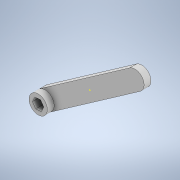
# Autodesk Inventor part: part
Saved by Autodesk Inventor 2020.2 (Build 242310000, 310)
## iProperties
Created: 2020-02-14
Part Number: part
Material: Generic
Document SubType Name: Modeling
Designer: robst
Density: 1 g/cm^3
Appearance: Default
Author: robst
Autodesk Inventor part; units mm, degrees
ref_plane "YZ Plane" through (0, 0, 0) normal (1, 0, 0) x (0, 1, 0)
ref_plane "XZ Plane" through (0, 0, 0) normal (0, 1, 0) x (-1, 0, 0)
ref_plane "XY Plane" through (0, 0, 0) normal (0, 0, 1) x (1, 0, 0)
sketch "Sketch1" plane through (0, 0, 0) normal (0, 0, 1) x (1, 0, 0)
  line L0 (-65.5382, -61.3942) -> (80.107, 40.5877)
  line L1 (80.107, 40.5877) -> (65.5382, 61.3942)
  line L2 (65.5382, 61.3942) -> (-80.107, -40.5877)
  line L3 (-80.107, -40.5877) -> (-65.5382, -61.3942)
  line L4 (-65.5382, -61.3942) -> (65.5382, 61.3942) construction
  line L5 (80.107, 40.5877) -> (-80.107, -40.5877) construction
  line L6 (-65.5382, -61.3942) -> (112.2618, -61.3942) construction
  point P0 (0, 0)
  dimension "d0" = 177.8
  dimension "d1" = 35
  dimension "d2" = 25.4
  constraints: 14 end point, 2 midpoint, 2 parallel, 1 equal length, 1 horizontal, 1 perpendicular
  measures "d0" distance of L0.start L0.end
  measures "d1" angle of L6 L0
  measures "d2" distance of L1.end L0.end
extrude "Extrusion1" add sketch "Sketch1" along normal blind 9.525
sketch "Sketch2" plane through (0, 0, 9.525) normal (0, 0, 1) x (1, 0, 0)
  point P0 (0, 0)
fillet "Fillet1" radius 12.7 4 edges at (65.5382, 61.3942, 4.7625) (80.107, 40.5877, 4.7625) (-65.5382, -61.3942, 4.7625) (-80.107, -40.5877, 4.7625)
sketch "Sketch3" plane through (0, 0, 9.525) normal (0, 0, 1) x (1, 0, 0)
  arc A0 (-69.7038, -33.3033) -> (-55.135, -54.1098) centre (-62.4194, -43.7065) ccw construction
  line L0 (-54.5275, -43.0212) -> (-57.88, -50.1984)
  line L1 (-57.88, -50.1984) -> (-65.7718, -50.8837)
  line L2 (-65.7718, -50.8837) -> (-70.3112, -44.3918)
  line L3 (-70.3112, -44.3918) -> (-66.9588, -37.2146)
  line L4 (-66.9588, -37.2146) -> (-59.0669, -36.5293)
  line L5 (-59.0669, -36.5293) -> (-54.5275, -43.0212)
  point P0 (0, 0)
  constraints: 12 end point, 1 coincident, 13 other
sketch "Sketch4" plane through (0, 0, 9.525) normal (0, 0, 1) x (1, 0, 0)
  arc A0 (-69.7038, -33.3033) -> (-55.135, -54.1098) centre (-62.4194, -43.7065) ccw projected
  line L0 (55.135, 54.1098) -> (-69.7038, -33.3033) projected
  circle A1 centre (-62.4194, -43.7065) radius 12.7
  point P0 (0, 0)
  point P1 (-55.135, -54.1098)
  constraints: 1 coincident, 3 other
extrude "Extrusion2" add sketch "Sketch4" along normal blind 9.525
extrude "Extrusion3" cut sketch "Sketch3" against normal mid plane 25.4
body "Solid1"
